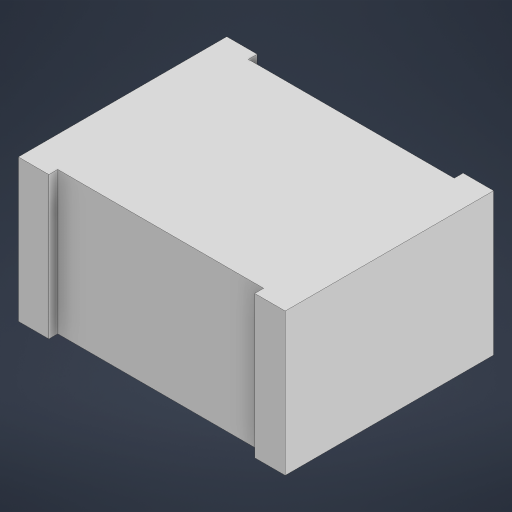
# Autodesk Inventor part: Magnet
Saved by Autodesk Inventor 2024.3 (Build 283343000, 343)
## iProperties
Created: 2024-06-12
Part Number: Magnet
Material: Generic
Document SubType Name: Modeling
Designer: braed
Density: 1 g/cm^3
Appearance: Default
Author: braed
Autodesk Inventor part; units mm, degrees
ref_plane "YZ Plane" through (0, 0, 0) normal (1, 0, 0) x (0, 1, 0)
ref_plane "XZ Plane" through (0, 0, 0) normal (0, 1, 0) x (-1, 0, 0)
ref_plane "XY Plane" through (0, 0, 0) normal (0, 0, 1) x (1, 0, 0)
sketch "Sketch1" plane through (0, 0, 0) normal (0, 0, 1) x (1, 0, 0)
  line L0 (0, 0) -> (166.6875, 0)
  line L1 (166.6875, 0) -> (166.6875, 130.175)
  line L2 (166.6875, 130.175) -> (0, 130.175)
  line L3 (0, 130.175) -> (0, 0)
  dimension "d0" = 166.6875
  dimension "d1" = 130.175
  constraints: 8 end point, 2 parallel, 1 horizontal, 1 perpendicular
  measures "d0" distance of L2.end L1.end
  measures "d1" distance of L1.end L0.end
extrude "Extrusion1" add sketch "Sketch1" along normal blind 88.9
sketch "Sketch3" plane through (0, 0, 0) normal (0, 0, -1) x (-1, 0, 0)
  line L0 (-166.6875, 0) -> (-166.6875, 130.175) construction
  line L1 (0, 0) -> (-166.6875, 0) projected
  line L2 (0, 130.175) -> (0, 0) construction
  line L3 (-166.6875, 130.175) -> (0, 130.175) construction
  line L4 (-166.6875, 0) -> (-147.6375, 0) construction
  line L5 (-147.6375, 0) -> (-147.6375, 5.5563)
  line L6 (0, 0) -> (-166.6875, 0) construction
  line L7 (-83.3438, 0) -> (-83.3438, 30.0341) construction
  line L8 (-166.6875, 0) -> (0, 0) construction
  line L9 (0, 0) -> (-19.05, 0) construction
  line L10 (-19.05, 0) -> (-19.05, 5.5563)
  line L11 (-166.6875, 0) -> (0, 0) construction
  line L12 (-19.05, 5.5563) -> (-147.6375, 5.5563)
  line L13 (-147.6375, 5.5563) -> (-19.05, 5.5563)
  line L14 (-19.05, 5.5563) -> (-19.05, 0)
  line L15 (-19.05, 0) -> (-147.6375, 0)
  line L16 (-147.6375, 0) -> (-147.6375, 5.5563)
  line L17 (-166.6875, 65.0875) -> (-112.8864, 65.0875) construction
  line L18 (-147.6375, 130.175) -> (-147.6375, 124.6187)
  line L19 (-19.05, 130.175) -> (-19.05, 124.6187)
  line L20 (-19.05, 124.6187) -> (-147.6375, 124.6187)
  line L21 (-147.6375, 124.6187) -> (-19.05, 124.6187)
  line L22 (-19.05, 124.6187) -> (-19.05, 130.175)
  line L23 (-19.05, 130.175) -> (-147.6375, 130.175)
  line L24 (-147.6375, 130.175) -> (-147.6375, 124.6187)
  point P0 (-83.3438, 130.175)
  constraints: 40 end point, 12 symmetric about line, 3 horizontal, 2 midpoint, 2 parallel, 2 perpendicular, 2 point on line, 1 vertical
extrude "Extrusion2" cut sketch "Sketch3" against normal through all
body "Solid1"
